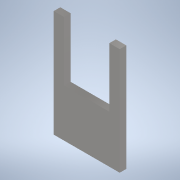
# Autodesk Inventor part: BackWheelMotorMountSpacer
Saved by Autodesk Inventor 2022.2 (Build 262287010, 287A)
## iProperties
Created: 2022-04-05
Part Number: BackWheelMotorMountSpacer
Material: Steel, Mild
Document SubType Name: Sheet Metal
Designer: Finn Oriwohl
Density: 7.85 g/cm^3
Sheet Metal Rule: Default_mm
Appearance: Semi-Polished
Author: Finn Oriwohl
Autodesk Inventor part; units mm, degrees
ref_plane "YZ Plane" through (0, 0, 0) normal (1, 0, 0) x (0, 1, 0)
ref_plane "XZ Plane" through (0, 0, 0) normal (0, 1, 0) x (-1, 0, 0)
ref_plane "XY Plane" through (0, 0, 0) normal (0, 0, 1) x (1, 0, 0)
sketch "Sketch1" plane through (0, 0, 0) normal (0, 0, 1) x (1, 0, 0)
  line L0 (113.6513, 30) -> (113.6513, 12) projected
  line L1 (113.6513, 12) -> (99.9513, 12) projected
  line L2 (99.9513, 12) -> (99.9513, 30) projected
  line L3 (99.9513, 30) -> (99.8013, 30) projected
  line L4 (99.8013, -3.4599) -> (99.8013, 30) projected
  line L5 (113.8013, -3.4599) -> (99.8013, -3.4599) projected
  line L6 (113.8013, 30) -> (113.8013, -3.4599) projected
  line L7 (113.8013, 30) -> (113.6513, 30) projected
  line L8 (96.8013, 30) -> (96.8013, -2.4219) projected
  line L9 (116.8013, 30) -> (116.8013, -2.4219) projected
  line L10 (116.8013, -2.4219) -> (96.8013, -2.4219)
  line L11 (96.8013, 30) -> (99.8013, 30)
  line L12 (113.8013, 30) -> (116.8013, 30)
  point P0 (0, 0)
  point P1 (99.8013, -2.4219)
  point P2 (113.8013, -2.4219)
  constraints: 6 end point, 2 point on line, 1 parallel, 1 other
extrude "Extrusion1" add sketch "Sketch1" along normal blind 2 contours L7 L6 L10 L4 L3 L2 L1 L0 | L12 L9 L10 L6 | L10 L8 L11 L4
equation "\"BendRadius\" = Thickness"
equation "\"BendReliefWidth\" = Thickness"
equation "\"BendReliefDepth\" = 0.5 * Thickness"
equation "\"CornerReliefSize\" = 4 * Thickness"
equation "\"MinimumRemnant\" = 2 * Thickness"
equation "\"TransitionRadius\" = BendRadius"
equation "\"JacobiRadiusSize\" = BendRadius"
equation "\"GapSize\" = Thickness"
equation "\"Thickness\" = 2"
body "Solid1"
